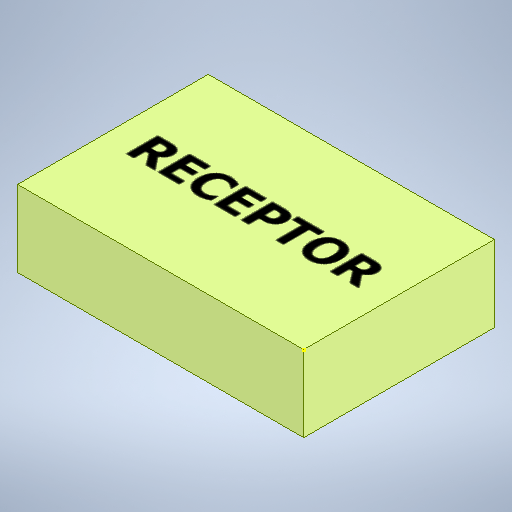
# Autodesk Inventor part: RECEPTOR
Saved by Autodesk Inventor 2025.3 (Build 293356030, 356C)
## iProperties
Created: 2025-07-08
Part Number: RECEPTOR
Material: Generic
Document SubType Name: Modeling
Designer: jv
Density: 1 g/cm^3
Appearance: Default(1)
Author: jv
Autodesk Inventor part; units mm, degrees
ref_plane "YZ Plane" through (0, 0, 0) normal (1, 0, 0) x (0, 1, 0)
ref_plane "XZ Plane" through (0, 0, 0) normal (0, 1, 0) x (-1, 0, 0)
ref_plane "XY Plane" through (0, 0, 0) normal (0, 0, 1) x (1, 0, 0)
sketch "Sketch1" plane through (0, 0, 0) normal (0, 1, 0) x (-1, 0, 0)
  line L0 (0, 0) -> (45, 0)
  line L1 (45, 0) -> (45, -30)
  line L2 (45, -30) -> (0, -30)
  line L3 (0, -30) -> (0, 0)
  dimension "d0" = 30
  dimension "d1" = 45
  constraints: 8 end point, 2 parallel, 1 horizontal, 1 perpendicular
  measures "d0" distance of L2.end L0.start
  measures "d1" distance of L1.end L2.end
extrude "Extrusion1" add sketch "Sketch1" along normal blind 12
sketch "Sketch2" plane through (0, 12, 0) normal (0, 1, 0) x (1, 0, 0)
  line L0 (-41.0785, 26.5716) -> (-4.1917, 26.5716) construction
  line L1 (-4.1917, 26.5716) -> (-4.1917, 3.8272) construction
  line L2 (-4.1917, 3.8272) -> (-41.0785, 3.8272) construction
  line L3 (-41.0785, 3.8272) -> (-41.0785, 26.5716) construction
  point P0 (0, 0)
  constraints: 2 other
body "Solid1"
